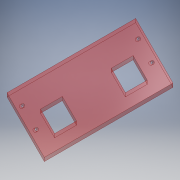
# Autodesk Inventor part: Front
Saved by Autodesk Inventor 2017 (Build 210142000, 142)
## iProperties
Created: 2016-11-10
Part Number: Front
Material: Generic
Document SubType Name: Modeling
Designer: Shichi
Density: 1 g/cm^3
Appearance: Dark Red
Author: Shichi
Autodesk Inventor part; units mm, degrees
ref_plane "YZ Plane" through (0, 0, 0) normal (1, 0, 0) x (0, 1, 0)
ref_plane "XZ Plane" through (0, 0, 0) normal (0, 1, 0) x (-1, 0, 0)
ref_plane "XY Plane" through (0, 0, 0) normal (0, 0, 1) x (1, 0, 0)
sketch "Sketch1" plane through (0, 0, 0) normal (0, 1, 0) x (-1, 0, 0)
  line L0 (0, 0) -> (0, -2.8284)
  line L1 (0, -2.8284) -> (29, 26.1716)
  line L2 (29, 26.1716) -> (29, 29)
  line L3 (29, 29) -> (0, 0)
  dimension "d2" = 29
  dimension "d3" = 45
  dimension "d6" = 2
  constraints: 8 end point, 1 parallel, 1 vertical
  measures "d2" horizontal distance of L0.end L1.end
  measures "d3" angle of L0 L1
  measures "d6" distance between parallel lines of L1 L3
extrude "Extrusion1" add sketch "Sketch1" along normal mid plane 100
sketch "Sketch2" plane through (0, 0, 0) normal (0, 0, 1) x (1, 0, 0)
  line L0 (-17, 36) -> (-6, 36)
  line L1 (-6, 36) -> (-6, 19)
  line L2 (-6, 19) -> (-17, 19)
  line L3 (-17, 19) -> (-17, 36)
  line L4 (0, 50) -> (-29, 50) projected
  line L5 (0, -50) -> (0, 50) projected
  point P0 (0, 0)
  dimension "d7" = 14
  dimension "d8" = 17
  dimension "d9" = 11
  dimension "d11" = 6
  constraints: 8 end point, 2 parallel, 1 horizontal, 1 perpendicular
  measures "d7" distance from line of L4 L0.start
  measures "d8" distance of L2.end L0.start
  measures "d9" distance of L1.end L2.end
  measures "d11" distance from line of L5 L0.end
extrude "Extrusion2" cut sketch "Sketch2" along normal up to next
mirror "Mirror1" about plane through (0, 0, 0) normal (0, 1, 0) of "Extrusion2"
sketch "Sketch3" plane through (0, -50, 0) normal (0.7071, 0, 0.7071) x (0.7071, 0, -0.7071)
  circle A0 centre (-30.5122, 5) radius 1.25
  circle A1 centre (-15.5122, 5) radius 1.25
  line L0 (-39.0122, 0) -> (-39.0122, 100) projected
  line L1 (-41.0122, 0) -> (-41.0122, 100) projected
  line L2 (0, 0) -> (-41.0122, 0) projected
  point P0 (0, 50)
  dimension "d15" = 5
  dimension "d16" = 2.5
  dimension "d17" = 15
  dimension "d18" = 2.5
  dimension "d19" = 5
  dimension "d20" = 10.5
  constraints: 2 centre point
  measures "d15" distance from line of L2 A0.centre
  measures "d16" diameter of A0
  measures "d17" distance of A1.centre A0.centre
  measures "d18" diameter of A1
  measures "d19" distance from line of L2 A1.centre
  measures "d20" distance from line of A0.centre L1
extrude "Extrusion3" cut sketch "Sketch3" against normal up to next
mirror "Mirror2" about plane through (0, 0, 0) normal (0, 1, 0) of "Extrusion3"
body "Solid1"
